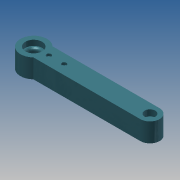
# Autodesk Inventor part: driven arm
Saved by Autodesk Inventor 2013 (Build 170138000, 138)
## iProperties
Created: 2017-03-30
Part Number: driven arm
Material: Generic
Document SubType Name: Modeling
Designer: employee
Density: 1 g/cm^3
Author: employee
Autodesk Inventor part; units mm, degrees
ref_plane "YZ Plane" through (0, 0, 0) normal (1, 0, 0) x (0, 1, 0)
ref_plane "XZ Plane" through (0, 0, 0) normal (0, 1, 0) x (-1, 0, 0)
ref_plane "XY Plane" through (0, 0, 0) normal (0, 0, 1) x (1, 0, 0)
sketch "Sketch1" plane through (0, 0, 0) normal (0, 0, 1) x (1, 0, 0)
  line L0 (0, 12.6) -> (153, 12.6)
  arc A0 (153, -12.6) -> (153, 12.6) centre (153, 0) ccw
  line L1 (153, -12.6) -> (0, -12.6)
  arc A1 (0, 12.6) -> (0, -12.6) centre (0, 0) ccw
  circle A2 centre (0, 0) radius 7.5
  circle A3 centre (153, 0) radius 4.25
  dimension "d0" = 153
  dimension "d2" = 12.6
  dimension "d3" = 15
  dimension "d4" = 8.5
  constraints: 4 centre point, 4 end point, 4 point on circle, 4 tangent, 3 coincident, 1 horizontal, 1 parallel
  measures "d0" distance of L0.start L0.end
  measures "d2" radius of A1
  measures "d3" diameter of A2
  measures "d4" diameter of A3
extrude "Extrusion1" add sketch "Sketch1" along normal blind 25
sketch "Sketch2" plane through (0, 0, 25) normal (0, 0, 1) x (1, 0, 0)
  circle A0 centre (0, 0) radius 7.5 projected
  arc A1 (0, 12.6) -> (0, -12.6) centre (0, 0) ccw projected
  circle A2 centre (0, 0) radius 11
  dimension "d7" = 22
  constraints: 1 centre point, 1 coincident
  measures "d7" diameter of A2
extrude "Extrusion2" cut sketch "Sketch2" against normal blind 7
sketch "Sketch4" plane through (0, 0, 25) normal (0, 0, 1) x (1, 0, 0)
  circle A0 centre (0, 0) radius 11 projected
  circle A1 centre (20, 0) radius 1.75
  circle A2 centre (40, 0) radius 1.75
  dimension "d16" = 20
  dimension "d17" = 40
  dimension "d23" = 3.5
  constraints: 2 centre point, 2 horizontal alignment, 1 equal radius
  measures "d16" distance of A1.centre A0.centre
  measures "d17" distance of A2.centre A0.centre
  measures "d23" diameter of A1
extrude "Extrusion3" cut sketch "Sketch4" against normal through all contours A1 | A2
sketch "Sketch5" plane through (0, 0, 25) normal (0, 0, 1) x (1, 0, 0)
  circle A0 centre (20, 0) radius 1.75 projected
  circle A1 centre (40, 0) radius 1.75 projected
  circle A2 centre (40, 0) radius 3
  circle A3 centre (20, 0) radius 3
  dimension "d28" = 6
  constraints: 2 centre point, 2 coincident, 1 equal radius
  measures "d28" diameter of A3
extrude "Extrusion4" cut sketch "Sketch5" against normal blind 3
sketch "Sketch6" plane through (0, 0, 25) normal (0, 0, 1) x (1, 0, 0)
  line L0 (153, 12.6) -> (0, 12.6) projected
  arc A0 (0, 12.6) -> (0, -12.6) centre (0, 0) ccw projected
  line L1 (0, -12.6) -> (153, -12.6) projected
  arc A1 (12.1445, 12.6) -> (12.1445, -12.6) centre (0, 0) ccw
  dimension "d24" = 35
  constraints: 2 point on circle, 2 point on line, 1 centre point, 1 coincident
  measures "d24" diameter of A1
extrude "Extrusion5" add sketch "Sketch6" against normal up to surface (25 mm away)
sketch "Sketch7" plane through (0, 0, 25) normal (0, 0, 1) x (1, 0, 0)
  circle A0 centre (153, 0) radius 4.25 projected
  arc A1 (153, -12.6) -> (153, 12.6) centre (153, 0) ccw projected
  circle A2 centre (153, 0) radius 7
  dimension "d30" = 14
  constraints: 1 centre point, 1 coincident
  measures "d30" diameter of A2
extrude "Extrusion6" cut sketch "Sketch7" against normal blind 8
fillet "Fillet1" radius 3.5 1 edges at (-7.5, 0, 18)
body "Solid1"
